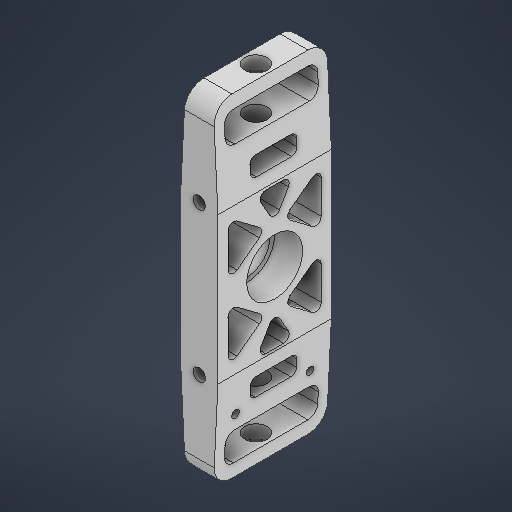
# Autodesk Inventor part: Front Upright
Saved by Autodesk Inventor 2026.1 (Build 301233000, 233)
## iProperties
Created: 2026-06-18
Part Number: Front Upright
Material: Generic
Document SubType Name: Modeling
Designer: share
Density: 1 g/cm^3
Appearance: Default
Author: share
Autodesk Inventor part; units mm, degrees
ref_plane "YZ Plane" through (0, 0, 0) normal (1, 0, 0) x (0, 1, 0)
ref_plane "XZ Plane" through (0, 0, 0) normal (0, 1, 0) x (-1, 0, 0)
ref_plane "XY Plane" through (0, 0, 0) normal (0, 0, 1) x (1, 0, 0)
sketch "Sketch1" plane through (0, 0, 0) normal (1, 0, 0) x (0, 1, 0)
  line L0 (-74.2701, 10.438) -> (74.2701, -10.438) construction
  line L1 (0, 42.6132) -> (0, -42.6132) construction
  line L2 (-131.9781, 0) -> (131.9781, 0) construction
  line L3 (-89.2701, -30.438) -> (89.2701, -30.438)
  line L4 (89.2701, -30.438) -> (89.2701, 30.438)
  line L5 (89.2701, 30.438) -> (-89.2701, 30.438)
  line L6 (-89.2701, 30.438) -> (-89.2701, -30.438)
  line L7 (74.2701, -10.438) -> (74.2701, 10.438) construction
  line L8 (74.2701, 10.438) -> (-74.2701, 10.438) construction
  line L9 (-74.2701, 10.438) -> (-74.2701, -10.438) construction
  line L10 (-74.2701, -10.438) -> (74.2701, -10.438) construction
  point P0 (0, 0)
  dimension "d1" = 150
  dimension "d8" = 8
  dimension "d11" = 20
  dimension "d12" = 15
  constraints: 18 end point, 3 parallel, 2 perpendicular, 2 vertical, 1 horizontal, 1 midpoint, 2 other
  measures "d1" distance of L0.start L0.end
  measures "d8" angle of L0 L2
  measures "d11" distance between parallel lines of L3 L10
  measures "d12" distance between parallel lines of L4 L7
extrude "Main Body" add sketch "Sketch1" along normal blind 10 and the other way blind 10
sketch "Sketch2" plane through (10, 0, 0) normal (1, 0, 0) x (0, 0, -1)
  line L0 (-10.438, -74.2701) -> (10.438, 74.2701) construction
  line L1 (-10.438, 74.2701) -> (-10.438, -74.2701) construction
  line L2 (-10.438, -74.2701) -> (10.438, -74.2701) construction
  line L3 (10.438, -74.2701) -> (10.438, 74.2701) construction
  line L4 (-42.6132, 0) -> (42.6132, 0) construction
  line L5 (0, -124.9781) -> (0, 124.9781) construction
  line L6 (10.438, 74.2701) -> (-10.438, 74.2701) construction
  line L7 (25, 66.3326) -> (-25, 66.3326)
  line L8 (-25, 66.3326) -> (-25, 82.2076)
  line L9 (-25, 82.2076) -> (25, 82.2076)
  line L10 (25, 82.2076) -> (25, 66.3326)
  line L11 (25, 66.3326) -> (-25, 82.2076) construction
  line L12 (-25, 66.3326) -> (25, 82.2076) construction
  line L13 (25, -66.3326) -> (-25, -66.3326)
  line L14 (-25, -66.3326) -> (-25, -82.2076)
  line L15 (-25, -82.2076) -> (25, -82.2076)
  line L16 (25, -82.2076) -> (25, -66.3326)
  line L17 (-12.5, 56.3326) -> (12.5, 56.3326)
  circle A0 centre (-20, -58.8326) radius 2.5
  circle A1 centre (20, -58.8326) radius 2.5
  line L18 (-12.5, 56.3326) -> (-12.5, 46.3326)
  line L19 (-12.5, 46.3326) -> (12.5, 46.3326)
  line L20 (12.5, 46.3326) -> (12.5, 56.3326)
  circle A2 centre (0, 0) radius 15
  line L21 (-12.5, -46.3326) -> (12.5, -46.3326)
  line L22 (12.5, -46.3326) -> (12.5, -56.3326)
  line L23 (12.5, -56.3326) -> (-12.5, -56.3326)
  line L24 (-12.5, -56.3326) -> (-12.5, -46.3326)
  circle A3 centre (0, 0) radius 12.5
  point P0 (0, 74.2701)
  dimension "d22" = 15.875
  dimension "d23" = 50
  dimension "d24" = 25
  dimension "d26" = 10
  dimension "d27" = 5
  dimension "d28" = 5
  dimension "d29" = 40
  dimension "d32" = 10
  dimension "d33" = 30
  dimension "d34" = 10
  dimension "d35" = 25
  dimension "d36" = 10
  dimension "d41" = 25
  constraints: 36 end point, 4 centre point, 4 parallel, 4 perpendicular, 4 symmetric about line, 3 horizontal, 3 midpoint, 2 coincident, 1 vertical, 3 other
  measures "d22" distance between parallel lines of L7 L9
  measures "d23" distance between parallel lines of L10 L8
  measures "d24" distance of L17.start L17.end
  measures "d26" distance between parallel lines of L17 L7
  measures "d27" diameter of A0
  measures "d28" distance edge to line of A0 L13
  measures "d29" distance of A1.centre A0.centre
  measures "d32" distance between parallel lines of L19 L17
  measures "d33" diameter of A2
  measures "d34" distance between parallel lines of L21 L23
  measures "d35" distance between parallel lines of L22 L24
  measures "d36" distance between parallel lines of L23 L13
  measures "d41" diameter of A3
extrude "Rod End Slots" cut sketch "Sketch2" against normal up to surface (20 mm away) contours L7 L8 L9 L10 | L16 L15 L14 L13 | L17 L20 L19 L18 | L21 L22 L23 L24
extrude "Axle Bore" cut sketch "Sketch2" against normal up to surface (20 mm away) contours A3
extrude "Wheel Bearing Bore" cut sketch "Sketch2" against normal blind 15 contours A2
hole "Toe Arm Holes" at (10, -58.8326, 20) at (10, -58.8326, -20) direction (-1, 0, 0) diameter 4.134 end through all thread size "M5x0.8" class "6H" standard "ISO Metric profile"
fillet "Rod End Slot Fillet" radius 5 8 edges at (0, 82.2076, 25) (0, 82.2076, -25) (0, 66.3326, 25) (0, 66.3326, -25) (0, -66.3326, 25) (0, -66.3326, -25) (0, -82.2076, -25) (0, -82.2076, 25)
fillet "Rod End Nut Slot Fillet" radius 3 8 edges at (0, 56.3326, 12.5) (0, 46.3326, 12.5) (0, 46.3326, -12.5) (0, 56.3326, -12.5) (0, -46.3326, -12.5) (0, -46.3326, 12.5) (0, -56.3326, 12.5) (0, -56.3326, -12.5)
sketch "Sketch3" plane through (-10, 89.2701, 30.438) normal (0, 1, 0) x (1, 0, 0)
  circle A0 centre (10, 30.438) radius 6
  dimension "d55" = 12
  constraints: 1 centre point, 1 coincident
  measures "d55" diameter of A0
sketch "Sketch4" plane through (-10, -89.2701, -30.438) normal (0, -1, 0) x (1, 0, 0)
  circle A0 centre (10, 30.438) radius 6 projected
extrude "Upper Rod End Bolt Hole" cut sketch "Sketch3" against normal up to surface (32.9375 mm away)
extrude "Lower Rod End Bolt Hole" cut sketch "Sketch4" against normal up to surface (32.9375 mm away)
sketch "Sketch5" plane through (-10, -89.2701, 30.438) normal (0, 0, 1) x (1, 0, 0)
  line L0 (0, 178.5402) -> (20, 178.5402) projected
  line L1 (10, 178.5402) -> (10, 0) construction
  line L2 (0, 0) -> (20, 0) projected
  line L3 (0, 0) -> (0, 178.5402) projected
  line L4 (0, 89.2701) -> (20, 89.2701) construction
  line L5 (20, 178.5402) -> (20, 0) projected
  point P0 (10, 89.2701)
  point P1 (10, 129.2701)
  point P2 (10, 49.2701)
  dimension "d60" = 80
  constraints: 4 end point, 4 midpoint, 2 point on line, 1 symmetric about line
  measures "d60" distance of point (10, 49.27) point (10, 129.27)
hole "Caliper Bracket Mounting Holes" at (0, 40, 30.438) at (0, -40, 30.438) direction (0, 0, -1) diameter 6.647 depth 10 tip angle 118 thread size "M8x1.25" class "6H" standard "ISO Metric profile"
sketch "Sketch6" plane through (10, 0, 0) normal (1, 0, 0) x (0, 0, -1)
  line L0 (-42.6132, 0) -> (42.6132, 0) construction
  line L1 (0, -124.9781) -> (0, 124.9781) construction
  line L2 (-25, 35) -> (-5, 20)
  line L3 (-5, 20) -> (-25, 5)
  line L4 (-25, 5) -> (-25, 35)
  line L5 (-5, 20) -> (-25, 20) construction
  line L6 (-25, -35) -> (-5, -20)
  line L7 (-5, -20) -> (-25, -5)
  line L8 (-25, -5) -> (-25, -35)
  line L9 (25, 35) -> (5, 20)
  line L10 (5, 20) -> (25, 5)
  line L11 (25, 5) -> (25, 35)
  line L12 (25, -35) -> (5, -20)
  line L13 (25, -5) -> (25, -35)
  line L14 (5, -20) -> (25, -5)
  line L15 (-10, 38) -> (10, 38)
  line L16 (10, 38) -> (0, 20.6795)
  line L17 (-10, 38) -> (0, 20.6795)
  line L18 (-10, -38) -> (10, -38)
  line L19 (10, -38) -> (0, -20.6795)
  line L20 (-10, -38) -> (0, -20.6795)
  point P0 (0, 0)
  dimension "d68" = 25
  dimension "d69" = 30
  dimension "d70" = 25
  dimension "d71" = 20
  dimension "d72" = 20
  dimension "d73" = 20
  dimension "d74" = 38
  constraints: 38 end point, 12 symmetric about line, 2 equal length, 1 horizontal, 1 midpoint, 1 parallel, 1 point on line, 1 vertical
  measures "d68" distance between parallel lines of L4 L1
  measures "d69" distance of L3.end L2.start
  measures "d70" distance of L2.start L2.end
  measures "d71" distance between parallel lines of L0 L5
  measures "d72" distance of L15.start L15.end
  measures "d73" distance of L15.end L16.end
  measures "d74" distance between parallel lines of L0 L15
extrude "Face Weight Reduction" cut sketch "Sketch6" against normal up to surface (20 mm away)
fillet "Weight Reduction Fillet" radius 3 18 edges at (0, 35, 25) (0, 20, 5) (0, 5, 25) (0, 38, -10) (0, 20.6795, 0) (0, 38, 10) (0, -5, -25) (0, -35, -25) (0, -20, -5) (0, -20, 5) (0, -35, 25) (0, -5, 25) (0, 20, -5) (0, 5, -25) (0, 35, -25) (0, -38, -10) (0, -38, 10) (0, -20.6795, 0)
sketch "Sketch7" plane through (-10, -89.2701, 30.438) normal (0, 0, 1) x (1, 0, 0)
  circle A0 centre (10, 49.2701) radius 3.3235 projected
  circle A1 centre (10, 129.2701) radius 3.3235 projected
  line L0 (0, 0) -> (20, 0) projected
  line L1 (20, 178.5402) -> (20, 0) projected
  line L2 (0, 178.5402) -> (20, 178.5402) projected
  line L3 (0, 0) -> (0, 178.5402) projected
  line L4 (0, 0) -> (0, 178.5402) construction
  line L5 (10, 214.2483) -> (10, -35.708) projected
  line L6 (-4, 89.2701) -> (24, 89.2701) projected
  line L7 (17.5, 0) -> (2.5, 0)
  line L8 (0, 89.2701) -> (0, 49.9375)
  line L9 (2.5, 0) -> (0, 49.9375)
  line L10 (17.5, 0) -> (20, 49.9375)
  line L11 (20, 49.9375) -> (20, 89.2701)
  line L12 (17.5, 178.5402) -> (2.5, 178.5402)
  line L13 (0, 89.2701) -> (0, 128.6027)
  line L14 (2.5, 178.5402) -> (0, 128.6027)
  line L15 (17.5, 178.5402) -> (20, 128.6027)
  line L16 (20, 128.6027) -> (20, 89.2701)
  point P0 (10, 89.2701)
  point P1 (10, 0)
  point P2 (20, 128.6027)
  point P3 (0, 128.6027)
  point P4 (20, 49.9375)
  point P5 (0, 49.9375)
  dimension "d85" = 15
  dimension "d86" = 50
  constraints: 20 end point, 5 symmetric about line, 4 midpoint, 4 point on line
  measures "d85" distance of L7.end L7.start
  measures "d86" distance of L7.end L8.end
extrude "Edge Weight Reduction" cut sketch "Sketch7" against normal up to surface (60.876 mm away) contours L0 L3 L9 | L10 L1 L0 | L3 L2 L14 | L15 L2 L1
fillet "Main Body Fillet" radius 10 4 edges at (0, -89.2701, -30.438) (0, -89.2701, 30.438) (0, 89.2701, -30.438) (0, 89.2701, 30.438)
equation "\"d1\" = Outboard_Point_Linear_Spacing"
equation "\"d8\" = Caster_Angle"
equation "\"d11\" = Upright_Width_From_UOP"
equation "\"d12\" = Upright_Height_From_UOP"
equation "\"d22\" = Rod_End_Slot_Height"
equation "\"d23\" = Rod_End_Slot_Width"
equation "\"d24\" = Upper_Rod_End_Bolt_Slot_Width"
equation "\"d26\" = Upper_Rod_End_Nut_Slot_Vertical_Spacing"
equation "\"d27\" = Toe_Arm_Hole_Diameter"
equation "\"d28\" = Toe_Arm_Hole_Vertical_Spacing"
equation "\"d29\" = Toe_Arm_Hole_Horizontal_Spacing"
equation "\"d32\" = Upper_Rod_End_Nut_Slot_Height"
equation "\"d33\" = Wheel_Bearing_Bore_Diameter"
equation "\"d34\" = Lower_Rod_End_Nut_Slot_Height"
equation "\"d35\" = Lower_Rod_End_Nut_Slot_Width"
equation "\"d36\" = Lower_Rod_End_Nut_Slot_Vertical_Spacing"
equation "\"d41\" = Axle_Bore_Diameter"
equation "\"d44\" = Wheel_Bearing_Bore_Depth"
equation "\"d47\" = Toe_Arm_Hole_Thread_Depth"
equation "\"d53\" = Rod_End_Slot_Fillet"
equation "\"d54\" = Rod_End_Nut_Slot_Fillet"
equation "\"d55\" = Rod_End_Bolt_Hole_Diameter"
equation "\"d60\" = Caliper_Bracket_Mount_Hole_Spacing"
equation "\"d62\" = Caliper_Bracket_Mount_Hole_Thread_Depth"
equation "\"d66\" = Caliper_Bracket_Mount_Hole_Depth"
equation "\"d77\" = Weight_Reduction_Fillet"
equation "\"Outboard_Point_Linear_Spacing\" = 150"
equation "\"Caster_Angle\" = 8deg"
equation "\"Upright_Width_From_UOP\" = 20"
equation "\"Upright_Height_From_UOP\" = 15"
equation "\"Rod_End_Slot_Height\" = 15.875"
equation "\"Rod_End_Slot_Width\" = 50"
equation "\"Toe_Arm_Hole_Diameter\" = 5"
equation "\"Toe_Arm_Hole_Vertical_Spacing\" = 5"
equation "\"Toe_Arm_Hole_Horizontal_Spacing\" = 40"
equation "\"Upper_Rod_End_Bolt_Slot_Width\" = 25"
equation "\"Upper_Rod_End_Nut_Slot_Height\" = 10"
equation "\"Lower_Rod_End_Nut_Slot_Width\" = 25"
equation "\"Lower_Rod_End_Nut_Slot_Height\" = 10"
equation "\"Lower_Rod_End_Nut_Slot_Vertical_Spacing\" = 10"
equation "\"Upper_Rod_End_Nut_Slot_Vertical_Spacing\" = 10"
equation "\"Wheel_Bearing_Bore_Diameter\" = 30"
equation "\"Toe_Arm_Hole_Depth\" = 8"
equation "\"Axle_Bore_Diameter\" = 25"
equation "\"Wheel_Bearing_Bore_Depth\" = 15"
equation "\"Toe_Arm_Hole_Thread_Depth\" = 6"
equation "\"Rod_End_Slot_Fillet\" = 5"
equation "\"Rod_End_Nut_Slot_Fillet\" = 3"
equation "\"Rod_End_Bolt_Hole_Diameter\" = 12"
equation "\"Caliper_Bracket_Mount_Hole_Spacing\" = 80"
equation "\"Caliper_Bracket_Mount_Hole_Depth\" = 10"
equation "\"Caliper_Bracket_Mount_Hole_Thread_Depth\" = 8"
equation "\"Weight_Reduction_Fillet\" = 3"
body "Solid1"
